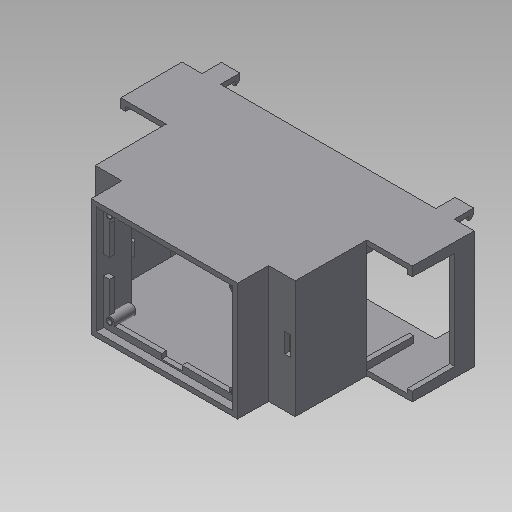
# Autodesk Inventor part: D2MG up
Saved by Autodesk Inventor 2018 (Build 220112000, 112)
## iProperties
Created: 2015-02-06
Part Number: D2MG up
Material: Типовые
Document SubType Name: Modeling
Designer: Abbath
Density: 1 g/cm^3
Appearance: По умолчанию
Mass: 16.1777 g
Surface Area: 228.387 cm^2
Volume: 16.1777 cm^3
Author: Abbath
Autodesk Inventor part; units mm, degrees
sketch "Эскиз1" plane through (0, 0, 0) normal (0, 1, 0) x (-1, 0, 0)
  line L0 (43.6, 0) -> (43.45, 19)
  line L1 (29.4899, 19) -> (29.3222, 39.5)
  line L2 (29.3222, 39.5) -> (21.151, 39.5)
  line L3 (21.151, 39.5) -> (21.07, 50.5)
  line L4 (-21.07, 50.5) -> (-21.151, 39.5)
  line L5 (-21.151, 39.5) -> (-29.3222, 39.5)
  line L6 (-29.3222, 39.5) -> (-29.4899, 19)
  line L7 (-43.45, 19) -> (-43.6, 0)
  line L8 (-43.6, 0) -> (-45.1, 0)
  line L9 (-45.1, 0) -> (-44.95, 19)
  line L10 (-44.95, 19) -> (-30.99, 19)
  line L11 (-30.99, 19) -> (-30.81, 41)
  line L12 (-30.81, 41) -> (-22.64, 41)
  line L13 (-22.64, 41) -> (-22.57, 50.5)
  line L14 (22.57, 50.5) -> (22.64, 41)
  line L15 (22.64, 41) -> (30.81, 41)
  line L16 (30.81, 41) -> (30.99, 19)
  line L17 (30.99, 19) -> (44.95, 19)
  line L18 (44.95, 19) -> (45.1, 0)
  line L19 (45.1, 0) -> (43.6, 0)
  line L20 (-30.99, 19) -> (-29.4899, 19)
  line L21 (30.99, 19) -> (29.4899, 19)
  line L22 (-22.57, 50.5) -> (-21.07, 50.5)
  line L23 (21.07, 50.5) -> (22.57, 50.5)
  line L24 (-30.99, 19) -> (-30.99, 13.4908) construction
  line L25 (30.99, 19) -> (30.99, 12.5683) construction
  point P0 (0, 0)
  dimension "d0" = 1.5
  dimension "d1" = 1.5
  dimension "d3" = 1.5
  dimension "d4" = 1.5
  dimension "d6" = 1.5
  dimension "d7" = 1.5
  dimension "d10" = 1.5
  dimension "d11" = 1.5
  dimension "d12" = 90.2
  dimension "d13" = 89.9
  dimension "d14" = 19
  dimension "d15" = 45.1
  dimension "d16" = 61.62
  dimension "d17" = 61.98
  dimension "d18" = 41
  dimension "d19" = 45.14
  dimension "d20" = 45.28
  dimension "d45" = 50.5
  constraints: 52 end point, 12 parallel, 6 equal length, 5 point on line, 4 horizontal, 2 collinear, 2 vertical
  measures "d0" distance between parallel lines of L0 L18
  measures "d1" distance between parallel lines of L1 L16
  measures "d3" distance between parallel lines of L2 L15
  measures "d4" distance between parallel lines of L3 L14
  measures "d6" distance between parallel lines of L13 L4
  measures "d7" distance between parallel lines of L5 L12
  measures "d10" distance between parallel lines of L9 L7
  measures "d11" distance between parallel lines of L11 L6
  measures "d12" distance of L8.end L18.end
  measures "d13" distance of L17.end L9.end
  measures "d14" distance between parallel lines of L17 L19
  measures "d15" distance of L18.end point (0, 0)
  measures "d16" distance of L11.end L15.end
  measures "d17" distance of L10.end L16.end
  measures "d18" distance between parallel lines of L15 L19
  measures "d19" distance of L13.end L14.start
  measures "d20" distance of L12.end L14.end
  measures "d45" distance from line of point (0, 0) L23
extrude "Выдавливание1" add sketch "Эскиз1" along normal mid plane 36.3
sketch "Эскиз10" plane through (0, -18.15, 0) normal (0, -1, 0) x (1, 0, 0)
  line L0 (-45.1, 0) -> (-44.95, 19)
  line L1 (-44.95, 19) -> (-30.99, 19)
  line L2 (-30.99, 19) -> (-30.81, 41)
  line L3 (-30.81, 41) -> (-22.64, 41)
  line L4 (-22.64, 41) -> (-22.57, 50.5)
  line L5 (-22.57, 50.5) -> (22.57, 50.5)
  line L6 (22.57, 50.5) -> (22.64, 41)
  line L7 (22.64, 41) -> (30.81, 41)
  line L8 (30.81, 41) -> (30.99, 19)
  line L9 (30.99, 19) -> (44.95, 19)
  line L10 (44.95, 19) -> (45.1, 0)
  line L11 (45.1, 0) -> (-45.1, 0)
  line L12 (22.57, 50.5) -> (-22.57, 50.5) construction
  line L13 (22.64, 41) -> (22.57, 50.5) construction
  line L14 (30.81, 41) -> (22.64, 41) construction
  line L15 (30.99, 19) -> (30.81, 41) construction
  line L16 (44.95, 19) -> (43.45, 19) construction
  line L17 (45.1, 0) -> (44.95, 19) construction
  line L18 (43.6, 0) -> (45.1, 0) construction
  line L19 (-44.95, 19) -> (-45.1, 0) construction
  line L20 (-43.45, 19) -> (-44.95, 19) construction
  line L21 (-30.81, 41) -> (-30.99, 19) construction
  line L22 (-22.64, 41) -> (-30.81, 41) construction
  line L23 (-22.57, 50.5) -> (-22.64, 41) construction
  point P0 (0, 0)
  constraints: 24 end point, 12 collinear, 5 parallel, 1 horizontal
extrude "Выдавливание2" add sketch "Эскиз10" against normal blind 1.5
sketch "Эскиз11" plane through (0, 18.15, 0) normal (0, 1, 0) x (1, 0, 0)
  line L0 (-45.1, 0) -> (45.1, 0) projected
  line L1 (45.1, 0) -> (44.95, -19) projected
  line L2 (44.95, -19) -> (30.99, -19) projected
  line L3 (30.99, -19) -> (30.81, -41) projected
  line L4 (30.81, -41) -> (22.64, -41) projected
  line L5 (22.64, -41) -> (22.57, -50.5) projected
  line L6 (22.57, -50.5) -> (-22.57, -50.5) projected
  line L7 (-22.57, -50.5) -> (-22.64, -41) projected
  line L8 (-22.64, -41) -> (-30.81, -41) projected
  line L9 (-30.81, -41) -> (-30.99, -19) projected
  line L10 (-30.99, -19) -> (-44.95, -19) projected
  line L11 (-44.95, -19) -> (-45.1, 0) projected
  point P0 (0, 0)
extrude "Выдавливание3" add sketch "Эскиз11" against normal blind 1.5
ref_plane "РабПлоскость6" through (45.1, 18.15, 46.7) normal (0, 0, -1) x (-1, 0, 0)
sketch "Эскиз12" plane through (45.1, 18.15, 46.7) normal (0, 0, -1) x (-1, 0, 0)
  line L0 (66.74, -35.3) -> (23.46, -35.3)
  line L1 (23.46, -1) -> (66.74, -1)
  line L2 (0, 0) -> (90.2, 0) construction
  line L3 (90.2, -36.3) -> (0, -36.3) construction
  line L4 (67.74, -36.3) -> (67.74, 0) construction
  line L5 (22.46, -36.3) -> (22.46, 0) construction
  line L6 (14.29, -36.3) -> (22.46, -36.3) construction
  line L7 (14.29, -36.3) -> (14.29, 0) construction
  line L8 (22.46, 0) -> (14.29, 0) construction
  line L9 (66.74, -21.05) -> (64.35, -21.05)
  line L10 (64.35, -21.05) -> (64.35, -30.7)
  line L11 (62.8301, -32.8) -> (48.25, -32.8)
  line L12 (48.25, -32.8) -> (48.25, -34.3)
  line L13 (48.25, -34.3) -> (41.95, -34.3)
  line L14 (41.95, -34.3) -> (41.95, -32.8)
  line L15 (41.95, -32.8) -> (27.3699, -32.8)
  line L16 (25.85, -30.7) -> (25.85, -21.05)
  line L17 (25.85, -21.05) -> (23.46, -21.05)
  line L18 (64.35, -15.25) -> (64.35, -5.6)
  line L19 (62.8301, -3.5) -> (48.25, -3.5)
  line L20 (48.25, -3.5) -> (48.25, -2)
  line L21 (48.25, -2) -> (41.95, -2)
  line L22 (41.95, -2) -> (41.95, -3.5)
  line L23 (41.95, -3.5) -> (27.3699, -3.5)
  line L24 (25.85, -5.6) -> (25.85, -15.25)
  line L25 (25.85, -15.25) -> (23.46, -15.25)
  line L26 (23.46, -35.3) -> (23.46, -21.05)
  line L27 (23.46, -15.25) -> (23.46, -1)
  line L28 (66.74, -1) -> (66.74, -15.25)
  line L29 (66.74, -21.05) -> (66.74, -35.3)
  line L30 (66.74, -15.25) -> (64.35, -15.25)
  arc A0 (25.85, -5.6) -> (27.3699, -3.5) centre (25.85, -4) ccw
  arc A1 (27.3699, -32.8) -> (25.85, -30.7) centre (25.85, -32.3) ccw
  arc A2 (62.8301, -3.5) -> (64.35, -5.6) centre (64.35, -4) ccw
  arc A3 (64.35, -30.7) -> (62.8301, -32.8) centre (64.35, -32.3) ccw
  point P0 (45.1, -18.15)
  dimension "d47" = 1
  dimension "d49" = 1
  dimension "d52" = 1
  dimension "d53" = 1
  dimension "d54" = 5.8
  dimension "d55" = 2.9
  dimension "d56" = 38.5
  dimension "d57" = 19.25
  dimension "d58" = 6.3
  dimension "d59" = 3.15
  dimension "d60" = 29.3
  dimension "d61" = 14.65
  dimension "d62" = 32.3
  dimension "d63" = 16.15
  dimension "d67" = 1.6
  dimension "d138" = 28.3
  dimension "d139" = 14.15
  dimension "d140" = 38.5
  dimension "d141" = 19.25
  constraints: 48 end point, 16 perpendicular, 10 collinear, 8 point on circle, 5 horizontal, 5 parallel, 4 centre point, 3 equal radius, 2 horizontal alignment, 2 vertical alignment, 1 vertical
  measures "d47" distance between parallel lines of L1 L2
  measures "d49" distance between parallel lines of L0 L3
  measures "d52" distance between parallel lines of L28 L4
  measures "d53" distance between parallel lines of L5 L27
  measures "d54" distance between parallel lines of L30 L9
  measures "d55" distance from line of point (45.1, -18.15) L9
  measures "d56" distance between parallel lines of L24 L18
  measures "d57" distance from line of point (45.1, -18.15) L24
  measures "d58" distance between parallel lines of L22 L20
  measures "d59" distance from line of point (45.1, -18.15) L20
  measures "d60" distance between parallel lines of L23 L15
  measures "d61" distance from line of point (45.1, -18.15) L15
  measures "d62" distance between parallel lines of L21 L13
  measures "d63" distance from line of point (45.1, -18.15) L13
  measures "d67" radius of A2
  measures "d138" distance of A2.centre A3.centre
  measures "d139" vertical distance of point (45.1, -18.15) A3.centre
  measures "d140" distance of A0.centre A2.centre
  measures "d141" horizontal distance of point (45.1, -18.15) A2.centre
extrude "Выдавливание4" add sketch "Эскиз12" against normal blind 1.5
sketch "Эскиз13" plane through (45.1, 18.15, 46.7) normal (0, 0, -1) x (-1, 0, 0)
  arc A0 (27.3699, -32.8) -> (25.85, -30.7) centre (25.85, -32.3) ccw construction
  arc A1 (25.85, -5.6) -> (27.3699, -3.5) centre (25.85, -4) ccw construction
  arc A2 (62.8301, -3.5) -> (64.35, -5.6) centre (64.35, -4) ccw construction
  arc A3 (64.35, -30.7) -> (62.8301, -32.8) centre (64.35, -32.3) ccw construction
  circle A4 centre (64.35, -32.3) radius 1.6
  circle A5 centre (64.35, -4) radius 1.6
  circle A6 centre (25.85, -4) radius 1.6
  circle A7 centre (25.85, -32.3) radius 1.6
  point P0 (45.1, -18.15)
  constraints: 4 centre point, 4 coincident, 4 equal radius
extrude "Выдавливание5" add sketch "Эскиз13" along normal blind 5.1
sketch "Эскиз14" plane through (45.1, 18.15, 48.2) normal (0, 0, 1) x (1, 0, 0)
  circle A0 centre (-64.35, -4) radius 1
  circle A1 centre (-64.35, -32.3) radius 1
  circle A2 centre (-25.85, -4) radius 1
  circle A3 centre (-25.85, -32.3) radius 1
  line L0 (-25.85, -5.6) -> (-25.85, -15.25) construction
  line L1 (-25.85, -21.05) -> (-25.85, -30.7) construction
  line L2 (-64.35, -30.7) -> (-64.35, -21.05) construction
  line L3 (-64.35, -15.25) -> (-64.35, -5.6) construction
  point P0 (-45.1, -18.15)
  dimension "d70" = 28.3
  dimension "d71" = 14.15
  dimension "d72" = 2
  constraints: 4 centre point, 4 point on line, 3 equal radius, 2 horizontal alignment
  measures "d70" distance of A1.centre A0.centre
  measures "d71" vertical distance of point (-45.1, -18.15) A1.centre
  measures "d72" diameter of A2
extrude "Выдавливание6" add sketch "Эскиз14" along normal blind 0.1
sketch "Эскиз15" plane through (-19.25, 14.15, 48.3) normal (0, 0, 1) x (1, 0, 0)
  circle A0 centre (0, 0) radius 1 construction
  circle A1 centre (38.5, 0) radius 1 construction
  circle A2 centre (38.5, -28.3) radius 1 construction
  circle A3 centre (0, -28.3) radius 1 construction
  circle A4 centre (0, -28.3) radius 1.6 projected
  point P0 (19.25, -14.15)
  constraints: 4 coincident
hole "Отверстие2" at (-19.25, 14.15, 48.3) at (19.25, 14.15, 48.3) at (19.25, -14.15, 48.3) at (-19.25, -14.15, 48.3) direction (0, 0, -1) diameter 1.5 depth 6 tip angle 118
sketch "Эскиз16" plane through (22.64, -18.15, 41) normal (0, 0, 1) x (1, 0, 0)
  line L0 (-51.9622, 1.5) -> (-51.9622, 34.8) construction
  line L1 (6.6822, 1.5) -> (6.6822, 34.8) construction
  line L2 (-51.9622, 21.15) -> (-50.2622, 21.15)
  line L3 (-50.2622, 21.15) -> (-50.2622, 15.15)
  line L4 (-50.2622, 15.15) -> (-51.9622, 15.15)
  line L5 (-51.9622, 15.15) -> (-51.9622, 21.15)
  line L6 (4.9822, 21.15) -> (6.6822, 21.15)
  line L7 (6.6822, 21.15) -> (6.6822, 15.15)
  line L8 (6.6822, 15.15) -> (4.9822, 15.15)
  line L9 (4.9822, 15.15) -> (4.9822, 21.15)
  point P0 (-22.64, 18.15)
  point P1 (6.6822, 18.15)
  point P2 (-51.9622, 18.15)
  dimension "d93" = 1.7
  dimension "d94" = 6
  constraints: 16 end point, 4 parallel, 2 collinear, 2 equal length, 2 horizontal, 2 horizontal alignment, 2 midpoint, 2 perpendicular
  measures "d93" distance of L2.start L2.end
  measures "d94" distance of L2.end L3.end
extrude "Выдавливание7" cut sketch "Эскиз16" against normal through all
sketch "Эскиз17" plane through (0, 0, 0) normal (0, 1, 0) x (-1, 0, 0)
  line L0 (21.151, 39.5) -> (29.3222, 39.5) construction
  line L1 (21.098, 46.7) -> (21.151, 39.5) construction
  line L2 (29.3222, 39.5) -> (29.4899, 19) construction
  line L3 (-21.151, 39.5) -> (-21.098, 46.7) construction
  line L4 (-29.3222, 39.5) -> (-21.151, 39.5) construction
  line L5 (-29.4899, 19) -> (-29.3222, 39.5) construction
  line L6 (-29.3762, 32.9) -> (-29.4171, 27.9)
  line L7 (-29.4171, 27.9) -> (-28.3762, 32.9)
  line L8 (-28.3762, 32.9) -> (-29.3762, 32.9)
  line L9 (29.3762, 32.9) -> (29.4171, 27.9)
  line L10 (29.4171, 27.9) -> (28.3762, 32.9)
  line L11 (28.3762, 32.9) -> (29.3762, 32.9)
  line L12 (22.64, 38.5) -> (22.64, 39.5)
  line L13 (22.64, 39.5) -> (20.14, 39.5)
  line L14 (20.14, 39.5) -> (21.14, 38.5)
  line L15 (21.14, 38.5) -> (22.64, 38.5)
  line L16 (-22.64, 38.5) -> (-22.64, 39.5)
  line L17 (-22.64, 39.5) -> (-20.14, 39.5)
  line L18 (-20.14, 39.5) -> (-21.14, 38.5)
  line L19 (-21.14, 38.5) -> (-22.64, 38.5)
  line L20 (22.57, 50.5) -> (22.64, 41) construction
  line L21 (-22.64, 41) -> (-22.57, 50.5) construction
  line L22 (22.64, 41) -> (30.81, 41) construction
  point P0 (0, 0)
  dimension "d97" = 1
  dimension "d98" = 1.5
  dimension "d100" = 2.5
  dimension "d101" = 1
  dimension "d103" = 5
  dimension "d136" = 6.6
  constraints: 28 end point, 5 collinear, 5 equal length, 2 horizontal, 2 parallel, 2 perpendicular, 2 point on line, 2 vertical
  measures "d97" distance of L12.start L12.end
  measures "d98" distance of L14.end L12.start
  measures "d100" distance from line of L13.end L12
  measures "d101" distance of L7.end L6.start
  measures "d103" distance from line of L9.end L11
  measures "d136" distance between parallel lines of L11 L0
extrude "Выдавливание8" add sketch "Эскиз17" along normal mid plane 4
ref_plane "РабПлоскость8" through (0, 13.5, 0) normal (0, 1, 0) x (-1, 0, 0)
sketch "Эскиз18" plane through (0, 13.5, 0) normal (0, 1, 0) x (-1, 0, 0)
  line L0 (27.5, 39.5) -> (27.5, 35)
  line L1 (27.5, 39.5) -> (28.9, 39.5)
  line L2 (28.9, 39.5) -> (28.65, 35)
  line L3 (28.65, 35) -> (27.5, 35)
  line L4 (21.151, 39.5) -> (29.3222, 39.5) construction
  line L5 (27.5, 42.7165) -> (27.5, 25.8513) construction
  point P0 (0, 0)
  dimension "d108" = 4.5
  dimension "d109" = 2.3
  dimension "d110" = 2.8
  dimension "d112" = 27.5
  constraints: 10 end point, 2 collinear, 2 vertical, 1 horizontal, 1 parallel
  measures "d108" distance between parallel lines of L3 L1
  measures "d109" diameter of L2.end L0
  measures "d110" diameter of L1.end L0
  measures "d112" distance from line of point (0, 0) L5
revolve "Вращение1" add sketch "Эскиз18" angle 360 about axis through (-27.5, 13.5, 39.5) along (0, 0, -1)
mirror "Зеркальное отражение1" about plane through (0, 0, 0) normal (0, 1, 0) of "Вращение1"
mirror "Зеркальное отражение2" about plane through (0, 0, 0) normal (1, 0, 0) of "Вращение1", "Зеркальное отражение1"
sketch "Эскиз19" plane through (0, 0, 0) normal (1, 0, 0) x (0, 1, 0)
  line L0 (-16.65, 19) -> (16.65, 19) construction
  line L1 (-15.3, 19) -> (-15.1, 6)
  line L2 (-15.1, 6) -> (15.1, 6)
  line L3 (15.1, 6) -> (15.3, 19)
  line L4 (15.3, 19) -> (-15.3, 19)
  point P0 (0, 0)
  dimension "d114" = 6
  dimension "d115" = 30.6
  dimension "d116" = 30.2
  dimension "d117" = 15.3
  dimension "d118" = 15.1
  constraints: 8 end point, 1 collinear, 1 horizontal, 1 parallel
  measures "d114" distance from line of L2 point (0, 0)
  measures "d115" distance of L3.end L1.start
  measures "d116" distance of L1.end L2.end
  measures "d117" horizontal distance of point (0, 0) L1.start
  measures "d118" horizontal distance of point (0, 0) L1.end
extrude "Выдавливание9" cut sketch "Эскиз19" along normal through all both and the other way through all
ref_plane "РабПлоскость10" through (38.9, 0, 0) normal (1, 0, 0) x (0, 1, 0)
ref_plane "РабПлоскость9" through (45.1, 0, 0) normal (1, 0, 0) x (0, 1, 0)
sketch "Эскиз20" plane through (38.9, 0, 0) normal (1, 0, 0) x (0, 1, 0)
  line L0 (18.15, 0) -> (18.15, -6)
  line L1 (18.15, -6) -> (16.65, -6)
  line L2 (16.65, -6) -> (15.45, -5)
  line L3 (15.45, -5) -> (15.45, -4.5)
  line L4 (15.45, -4.5) -> (16.65, -4.5)
  line L5 (16.65, -4.5) -> (16.65, 0)
  line L6 (16.65, 0) -> (18.15, 0)
  line L7 (-18.15, 0) -> (-18.15, -6)
  line L8 (-18.15, -6) -> (-16.65, -6)
  line L9 (-16.65, -6) -> (-15.45, -5)
  line L10 (-15.45, -5) -> (-15.45, -4.5)
  line L11 (-15.45, -4.5) -> (-16.65, -4.5)
  line L12 (-16.65, -4.5) -> (-16.65, 0)
  line L13 (-16.65, 0) -> (-18.15, 0)
  point P0 (0, 0)
  point P1 (-16.65, 0)
  dimension "d123" = 6
  dimension "d124" = 0.5
  dimension "d125" = 1.5
  dimension "d126" = 2.7
  constraints: 28 end point, 7 perpendicular, 4 coincident, 2 collinear, 2 equal length, 2 parallel, 2 point on line, 2 vertical, 1 horizontal
  measures "d123" distance between parallel lines of L1 L6
  measures "d124" distance of L2.end L3.end
  measures "d125" distance between parallel lines of L1 L4
  measures "d126" distance from line of L3.end L0
extrude "Выдавливание10" add sketch "Эскиз20" against normal blind 5.7
mirror "Зеркальное отражение3" about plane through (0, 0, 0) normal (1, 0, 0) of "Выдавливание10"
ref_plane "РабПлоскость11" through (30.99, 0, 19) normal (1, 0, 0) x (0, 1, 0)
sketch "Эскиз21" plane through (30.99, 0, 19) normal (1, 0, 0) x (0, 1, 0)
  line L0 (-16.65, 0) -> (-16.65, -14.5)
  line L1 (-16.65, 0) -> (-16.65, -19) projected
  line L2 (-16.65, -14.5) -> (-14.75, -14.5)
  line L3 (-14.75, -14.5) -> (-14.45, 0)
  line L4 (-14.45, 0) -> (-16.65, 0)
  line L5 (16.65, 0) -> (16.65, -14.5)
  line L6 (16.65, -14.5) -> (14.75, -14.5)
  line L7 (14.75, -14.5) -> (14.45, 0)
  line L8 (14.45, 0) -> (16.65, 0)
  line L9 (-16.65, 0) -> (16.65, 0) construction
  line L10 (16.65, -19) -> (16.65, 0) construction
  point P0 (0, -19)
  dimension "d130" = 14.5
  dimension "d131" = 29.5
  dimension "d132" = 14.75
  dimension "d133" = 28.9
  constraints: 16 end point, 6 collinear, 2 parallel, 2 perpendicular, 1 equal length, 1 vertical
  measures "d130" distance between parallel lines of L2 L9
  measures "d131" distance of L6.end L2.end
  measures "d132" horizontal distance of point (0, -19) L2.end
  measures "d133" distance of L7.end L3.end
extrude "Выдавливание11" add sketch "Эскиз21" against normal blind 1.5
mirror "Зеркальное отражение4" about plane through (0, 0, 0) normal (1, 0, 0) of "Выдавливание11"
fillet "Сопряжение1" [suppressed]
equation "\"d1\" = d2"
equation "\"d3\" = d1"
equation "\"d4\" = d3"
equation "\"d6\" = d5"
equation "\"d7\" = d5"
equation "\"d10\" = d9"
equation "\"d11\" = d10"
equation "\"d15\" = 0.5 * d12"
equation "\"d55\" = 0.5 * d54"
equation "\"d57\" = 0.5 * d56"
equation "\"d59\" = 0.5 * d58"
equation "\"d61\" = 0.5 * d60"
equation "\"d63\" = 0.5 * d62"
equation "\"d71\" = 0.5 * d70"
equation "\"d2\" = d0"
equation "\"d5\" = d4"
equation "\"d9\" = d7"
